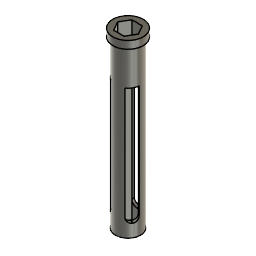
ALL+COMPONENTS+TOGETHER (Autodesk Fusion 360 archive; units mm, degrees)
design "pen holder"
part number: 2025-11-26-14-12-30-338
Autodesk Fusion 360 part; units mm, degrees
note: some values were not read from the file. Set by a fixed rule: which face or edge a step refers to.
sketch "Sketch1" plane through (0, 0, 0) normal (0, 0, 1) x (1, 0, 0)
  circle A0 centre (0, 0) radius 4.9
  line L0 (1.7696, -3.2108) -> (3.6654, -0.0729)
  line L1 (3.6654, -0.0729) -> (1.8959, 3.1379)
  line L2 (1.8959, 3.1379) -> (-1.7696, 3.2108)
  line L3 (-1.7696, 3.2108) -> (-3.6654, 0.0729)
  line L4 (-3.6654, 0.0729) -> (-1.8959, -3.1379)
  line L5 (-1.8959, -3.1379) -> (1.7696, -3.2108)
  dimension "d1" = 9.8
  dimension "d2" = 3.175
  constraint coincident A0.centre origin
  measures "d1" diameter of A0
  measures "d2" distance of A0.centre L5
extrude "Extrude1" add sketch "Sketch1" along normal blind 20 makes body 1
sketch "Sketch2" plane through (0, 0, 20) normal (0, 0, 1) x (-1, 0, 0)
  line L0 (-1.7696, 3.2108) -> (1.8959, 3.1379)
  line L1 (1.8959, 3.1379) -> (3.6654, -0.0729)
  line L2 (3.6654, -0.0729) -> (1.7696, -3.2108)
  line L3 (1.7696, -3.2108) -> (-1.8959, -3.1379)
  line L4 (-1.8959, -3.1379) -> (-3.6654, 0.0729)
  line L5 (-3.6654, 0.0729) -> (-1.7696, 3.2108)
  circle A0 centre (0, 0) radius 4.9
  circle A1 centre (0, 0) radius 6
  dimension "d6" = 12
  constraint concentric A0 A1
  measures "d6" diameter of A1
extrude "Extrude2" add sketch "Sketch2" against normal blind 3 contours A1 bodies 1
sketch "Sketch3" plane through (0, 0, 0) normal (0, 0, -1) x (1, 0, 0)
  line L0 (-1.8959, 3.1379) -> (1.7696, 3.2108)
  line L1 (1.7696, 3.2108) -> (3.6654, 0.0729)
  line L2 (3.6654, 0.0729) -> (1.8959, -3.1379)
  line L3 (1.8959, -3.1379) -> (-1.7696, -3.2108)
  line L4 (-1.7696, -3.2108) -> (-3.6654, -0.0729)
  line L5 (-3.6654, -0.0729) -> (-1.8959, 3.1379)
  circle A0 centre (0, 0) radius 4.9
sketch "Sketch4" plane through (0, 0, 20) normal (0, 0, 1) x (-1, 0, 0)
  circle A0 centre (0, 0) radius 6
  line L0 (-1.7696, 3.2108) -> (1.8959, 3.1379)
  line L1 (1.8959, 3.1379) -> (3.6654, -0.0729)
  line L2 (3.6654, -0.0729) -> (1.7696, -3.2108)
  line L3 (1.7696, -3.2108) -> (-1.8959, -3.1379)
  line L4 (-1.8959, -3.1379) -> (-3.6654, 0.0729)
  line L5 (-3.6654, 0.0729) -> (-1.7696, 3.2108)
  circle A1 centre (0, 0) radius 6
  line L6 (-2.0188, 3.5685) -> (-4.0998, 0.0359)
  line L7 (-4.0998, 0.0359) -> (-2.081, -3.5326)
  line L8 (-2.081, -3.5326) -> (2.0188, -3.5685)
  line L9 (2.0188, -3.5685) -> (4.0998, -0.0359)
  line L10 (4.0998, -0.0359) -> (2.081, 3.5326)
  line L11 (2.081, 3.5326) -> (-2.0188, 3.5685)
  dimension "d9" = 4.1
  constraint coincident A0.centre A1.centre
  measures "d9" distance of L6.start A0.centre
extrude "Extrude3" cut sketch "Sketch4" against normal blind 26 contours L6 L7 L8 L9 L10 L11 bodies 1
extrude "Extrude4" add 1 faces at (-0.1428, -3.9958, 0) along direction (0, 0, -1) blind 118 on bodies 1 bodies 1
extrude "Extrude5" cut 1 faces at (-0.1428, -3.9958, -118) along direction (0, 0, 1) blind 7 on bodies 1 bodies 1
extrude "Extrude6" cut 1 faces at (-0.1428, -3.9958, -111) along direction (0, 0, 1) blind 80 on bodies 1 bodies 1
sketch "Sketch5" plane through (0, 0, -31) normal (0, 0, -1) x (1, 0, 0)
  line L0 (2.0188, 3.5685) -> (4.0998, 0.0359)
  line L1 (4.0998, 0.0359) -> (2.081, -3.5326)
  line L2 (2.081, -3.5326) -> (-2.0188, -3.5685)
  line L3 (-2.0188, -3.5685) -> (-4.0998, -0.0359)
  line L4 (-4.0998, -0.0359) -> (-2.081, 3.5326)
  line L5 (-2.081, 3.5326) -> (2.0188, 3.5685)
  circle A0 centre (0, 0) radius 4.9
  circle A1 centre (0, 0) radius 4.9
  circle A2 centre (0, 0) radius 4.95
  dimension "d18" = 9.9
  constraint concentric A1 A2
  measures "d18" diameter of A2
extrude "Extrude7" add sketch "Sketch5" against normal blind 48 contours A2 bodies 1
extrude "Extrude8" add 1 faces at (3.5469, 1.8815, -31) along direction (0, 0, -1) blind 10 on bodies 1 bodies 1
ref_plane "WorkPlane1" through (0, 0, -37) normal (0, 0, -1) x (-1, 0, 0)
sketch "Sketch6" plane through (0, 0, -37) normal (0, 0, -1) x (-1, 0, 0)
  circle A0 centre (0, 0) radius 4.95
  line L0 (-2.0188, -3.5685) -> (-4.0998, -0.0359)
  line L1 (-4.0998, -0.0359) -> (-2.081, 3.5326)
  line L2 (-2.081, 3.5326) -> (2.0188, 3.5685)
  line L3 (2.0188, 3.5685) -> (4.0998, 0.0359)
  line L4 (4.0998, 0.0359) -> (2.081, -3.5326)
  line L5 (2.081, -3.5326) -> (-2.0188, -3.5685)
  line L6 (-2.081, 3.5326) -> (-2.0894, 4.4874)
  line L7 (2.0188, 3.5685) -> (2.0105, 4.5233)
  line L8 (4.0998, 0.0359) -> (4.9309, -0.4343)
  line L9 (2.081, -3.5326) -> (2.9121, -4.0028)
  line L10 (-2.0188, -3.5685) -> (-2.8416, -4.0532)
  line L11 (-4.0998, -0.0359) -> (-4.9226, -0.5205)
  line L12 (4.0998, 0.0359) -> (2.081, -3.5326)
  line L13 (2.081, -3.5326) -> (-2.0188, -3.5685)
  line L14 (2.0188, 3.5685) -> (4.0998, 0.0359)
  line L15 (-2.081, 3.5326) -> (2.0188, 3.5685)
  line L16 (-4.0998, -0.0359) -> (-2.081, 3.5326)
  line L17 (-2.0188, -3.5685) -> (-4.0998, -0.0359)
  circle A1 centre (0, 0) radius 4.95
  constraint coincident L1.end L2.start
  constraint coincident A0 L6.end
  constraint perpendicular L2 L6
  constraint coincident L2.end L3.start
  constraint coincident A0 L7.end
  constraint perpendicular L2 L7
  constraint coincident L3.end L4.start
  constraint coincident A0 L8.end
  constraint perpendicular L4 L8
  constraint coincident L4.end L5.start
  constraint coincident A0 L9.end
  constraint perpendicular L4 L9
  constraint coincident L0.start L5.end
  constraint coincident A0 L10.end
  constraint perpendicular L0 L10
  constraint coincident L0.end L1.start
  constraint coincident A0 L11.end
  constraint perpendicular L0 L11
split "Split1" by plane through (0, 0, -37) normal (0, 0, -1) bodies 1 makes body 2 at (4.9254, -0.4929, -38.3333)
extrude "Extrude9" cut sketch "Sketch6" against normal blind 40 contours A0 L2 L6 L7 L15 A1 | A0 L4 L8 L9 L12 A1 | A0 L0 L10 L11 L17 A1 bodies 1
move_body "Move1" bodies 2 to x (1, 0, 0) y (0, 1, 0) z (0, 0, 1) at (0, 0, -50)
extrude "Extrude10" add 3 faces at (0.0785, -4.0141, -37) (-3.4002, 2.1348, -37) (3.4516, 2.0525, -37) along direction (0, 0, -1) blind 5 on bodies 1 bodies 1
extrude "Extrude11" add 1 faces at (3.5469, 1.8815, -91) along direction (0, 0, -1) blind 1 on bodies 2 bodies 2
extrude "Extrude12" add 3 faces at (3.5489, 1.8772, -42) (0.0785, -4.0141, -42) (-3.4002, 2.1348, -42) along direction (0, 0, -1) blind 1 on bodies 1 bodies 1
move_body "Align1" bodies 1 to x (1, 0, 0) y (0, 1, 0) z (0, 0, 1) at (0, 0, -44)
combine "Combine1" operation add target body 2 tool bodies 1
fillet "Fillet1" radius 2 2 edges at (4.5112, -0.2782, -87) (2.4302, -3.8108, -87) on bodies 2
fillet "Fillet2" radius 2 4 edges at (-2.0147, 4.0459, -87) (2.0852, 4.01, -87) (-4.5154, -0.1992, -87) (-2.4965, -3.7677, -87) on bodies 2

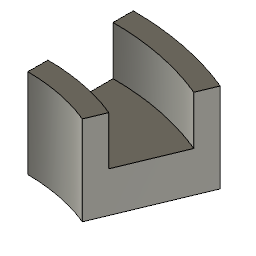
design "legs4"
part number: 2025-11-26-13-44-24-886
Autodesk Fusion 360 part; units mm, degrees
sketch "Sketch1" plane through (0, 0, 0) normal (0, 0, 1) x (1, 0, 0)
  circle A0 centre (0, 0) radius 48.975
  circle A1 centre (0, 0) radius 65.025
  circle A2 centre (0, 0) radius 70.025
  circle A3 centre (0, 0) radius 43.975
  dimension "d7" = 5
  dimension "d9" = -5
extrude "Extrude1" add sketch "Sketch1" along normal blind 12 makes body 1 at (48.9141, -2.4412, 8) makes body 2 at (69.938, -3.4905, 8)
sketch "Sketch2" plane through (0, 0, 0) normal (0, 0, 1) x (1, 0, 0)
  circle A0 centre (0, 0) radius 70
  constraint coincident A0.centre origin
extrude "Extrude2" add sketch "Sketch2" against normal blind 10 bodies 1 2
delete_face "DeleteFace1" 1 faces at (-13.2067, 6.36, 0) on bodies 1
split "Split1" by plane through (0, 0, 0) normal (1, 0, 0) bodies 1 makes body 3 at (60.9383, -5.4068, -10)
delete_body "RemoveBody1" bodies 3
move_body "Move1" bodies 1 to x (0.92388, -0.382683, 0) y (0.382683, 0.92388, 0) z (0, 0, 1) at (0, 0, 0)
split "Split2" by plane through (0, 0, 0) normal (1, 0, 0) bodies 1 makes body 4 at (12.8786, 59.8308, -10)
delete_body "RemoveBody2" bodies 1
equation "d8 = 5.00 mm"
equation "d9 = -d8"

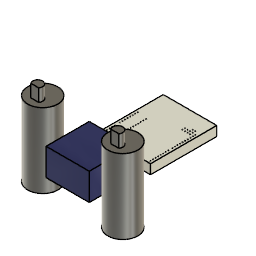
design "elec pieces"
part number: 2025-10-21-14-38-55-580
part number: 2025-10-21-14-53-44-347
part number: 2025-10-21-15-16-38-518
part number: 2025-10-21-15-29-22-499
Autodesk Fusion 360 part; units mm, degrees
sketch "Sketch1" plane through (0, 0, 0) normal (0, 0, 1) x (1, 0, 0)
sketch "Sketch2" plane through (0, -1.65, 0) normal (0, -1, 0) x (1, 0, 0)
  line L0 (0, -66.04) -> (0, 0)
  line L1 (0, 0) -> (-53.34, 0)
  line L2 (-53.34, 0) -> (-53.34, -66.04)
  line L3 (-53.34, -66.04) -> (-40.386, -66.04)
  line L4 (-40.386, -66.04) -> (-37.846, -68.58)
  line L5 (-37.846, -68.58) -> (-5.08, -68.58)
  line L6 (-5.08, -68.58) -> (-2.54, -66.04)
  line L7 (-2.54, -66.04) -> (0, -66.04)
  circle A0 centre (-2.54, -33.02) radius 0.4
  circle A1 centre (-2.54, -35.56) radius 0.4
  circle A2 centre (-2.54, -38.1) radius 0.4
  circle A3 centre (-2.54, -40.64) radius 0.4
  circle A4 centre (-2.54, -43.18) radius 0.4
  circle A5 centre (-2.54, -45.72) radius 0.4
  circle A6 centre (-2.54, -50.8) radius 0.4
  circle A7 centre (-2.54, -53.34) radius 0.4
  circle A8 centre (-2.54, -55.88) radius 0.4
  circle A9 centre (-2.54, -58.42) radius 0.4
  circle A10 centre (-2.54, -60.96) radius 0.4
  circle A11 centre (-2.54, -63.5) radius 0.4
  circle A12 centre (-50.8, -23.876) radius 0.4
  circle A13 centre (-50.8, -26.416) radius 0.4
  circle A14 centre (-50.8, -28.956) radius 0.4
  circle A15 centre (-50.8, -31.496) radius 0.4
  circle A16 centre (-50.8, -34.036) radius 0.4
  circle A17 centre (-50.8, -36.576) radius 0.4
  circle A18 centre (-50.8, -39.116) radius 0.4
  circle A19 centre (-50.8, -41.656) radius 0.4
  circle A20 centre (-50.8, -50.8) radius 0.4
  circle A21 centre (-50.8, -53.34) radius 0.4
  circle A22 centre (-50.8, -55.88) radius 0.4
  circle A23 centre (-50.8, -58.42) radius 0.4
  circle A24 centre (-50.8, -60.96) radius 0.4
  circle A25 centre (-50.8, -63.5) radius 0.4
  circle A26 centre (-12.573, -62.865) radius 0.4
  circle A27 centre (-20.193, -62.865) radius 0.4
  circle A28 centre (-12.573, -60.325) radius 0.4
  circle A29 centre (-20.193, -60.325) radius 0.4
  circle A30 centre (-12.573, -57.785) radius 0.4
  circle A31 centre (-20.193, -57.785) radius 0.4
  circle A32 centre (-12.573, -55.245) radius 0.4
  circle A33 centre (-20.193, -55.245) radius 0.4
  circle A34 centre (-12.573, -52.705) radius 0.4
  circle A35 centre (-20.193, -52.705) radius 0.4
  circle A36 centre (-12.573, -50.165) radius 0.4
  circle A37 centre (-20.193, -50.165) radius 0.4
  circle A38 centre (-12.573, -47.625) radius 0.4
  circle A39 centre (-20.193, -47.625) radius 0.4
  circle A40 centre (-12.573, -45.085) radius 0.4
  circle A41 centre (-20.193, -45.085) radius 0.4
  circle A42 centre (-12.573, -42.545) radius 0.4
  circle A43 centre (-20.193, -42.545) radius 0.4
  circle A44 centre (-12.573, -40.005) radius 0.4
  circle A45 centre (-20.193, -40.005) radius 0.4
  circle A46 centre (-12.573, -37.465) radius 0.4
  circle A47 centre (-20.193, -37.465) radius 0.4
  circle A48 centre (-12.573, -34.925) radius 0.4
  circle A49 centre (-20.193, -34.925) radius 0.4
  circle A50 centre (-12.573, -32.385) radius 0.4
  circle A51 centre (-20.193, -32.385) radius 0.4
  circle A52 centre (-12.573, -29.845) radius 0.4
  circle A53 centre (-20.193, -29.845) radius 0.4
  circle A54 centre (-26.162, -16.383) radius 0.5
  circle A55 centre (-26.162, -21.463) radius 0.5
  circle A56 centre (-39.878, -18.288) radius 0.4
  circle A57 centre (-39.878, -20.828) radius 0.4
  circle A58 centre (-42.418, -20.828) radius 0.4
  circle A59 centre (-42.418, -18.288) radius 0.4
  circle A60 centre (-44.958, -15.748) radius 0.4
  circle A61 centre (-44.958, -18.288) radius 0.4
  circle A62 centre (-44.958, -20.828) radius 0.4
  circle A63 centre (-47.498, -20.828) radius 0.4
  circle A64 centre (-47.498, -18.288) radius 0.4
  circle A65 centre (-47.498, -15.748) radius 0.4
  circle A66 centre (-30.43, -63.64) radius 0.4
  circle A67 centre (-27.89, -63.64) radius 0.4
  circle A68 centre (-25.35, -63.64) radius 0.4
  circle A69 centre (-25.35, -66.18) radius 0.4
  circle A70 centre (-27.89, -66.18) radius 0.4
  circle A71 centre (-30.43, -66.18) radius 0.4
  circle A72 centre (-50.8, -48.26) radius 0.4
  circle A73 centre (-50.8, -21.336) radius 0.4
  circle A74 centre (-50.8, -45.72) radius 0.4
  circle A75 centre (-2.54, -30.48) radius 0.4
  circle A76 centre (-50.8, -18.796) radius 0.4
  circle A77 centre (-2.54, -27.94) radius 0.4
  circle A78 centre (-50.8, -15.24) radius 1.5875
  circle A79 centre (-2.54, -13.97) radius 1.5875
  circle A80 centre (-35.56, -66.04) radius 1.5875
  circle A81 centre (-7.62, -66.04) radius 1.5875
  line L8 (-53.34, 0) -> (0, 0)
  line L9 (0, 0) -> (0, -66.04)
  line L10 (0, -66.04) -> (-53.34, -66.04)
  line L11 (-53.34, -66.04) -> (-53.34, 0)
  constraint horizontal L8
  constraint vertical L9
  constraint horizontal L10
  constraint vertical L11
  constraint coincident L0.start L7.end
  constraint coincident L1.end L2.start
extrude "Extrude1" add sketch "Sketch2" along normal blind 9.55 contours L0 L1 L2 L3 L7 A69 A70 A71 A80 A81 L8 L9 L10 L11 | A81 L10 | A80 L10 | A78 | A79 picked at (-7.5022, -65.5241) picked at (-35.4422, -65.5241) makes body 1 in component "Breadboard"
delete_face "DeleteFace1" 15 faces at (-25.6775, -8.0167, -21.5864) (-25.8129, -8.0167, -16.0251) (-20.183, -8.0167, -29.4451) (-19.7935, -8.0167, -32.4049) (-19.7935, -8.0167, -34.9449) (-19.7935, -8.0167, -37.4849) (-19.7935, -8.0167, -40.0249) (-19.7935, -8.0167, -42.5649) (-19.7935, -8.0167, -45.1049) (-19.7935, -8.0167, -47.6449) (-19.7935, -8.0167, -50.1849) (-19.7935, -8.0167, -52.7249) (-19.7935, -8.0167, -55.2649) (-19.7935, -8.0167, -57.8049) (-19.7935, -8.0167, -60.3449) on bodies 1 in component "Breadboard"
delete_face "DeleteFace2" 9 faces at (-25.0188, -8.0167, -65.9556) (-28.2212, -4.8333, -65.9556) (-30.7612, -4.8333, -65.9556) (-30.0305, -8.0167, -63.6599) (-27.4905, -8.0167, -63.6599) (-24.9505, -8.0167, -63.6599) (-19.7935, -8.0167, -62.8849) (-12.9143, -8.0167, -63.0736) (-12.9143, -8.0167, -60.5336) on bodies 1 in component "Breadboard"
sketch "Sketch3" plane through (0, 0, 0) normal (0, 1, 0) x (1, 0, 0)
  circle A0 centre (15, -15) radius 15
  dimension "d3" = 30
  measures "d3" diameter of A0
extrude "Extrude1'" add sketch "Sketch3" along normal blind 74.1 separate body makes body 2
sketch "Sketch4" plane through (0, 74.1, 0) normal (0, 1, 0) x (-1, 0, 0)
  circle A0 centre (-15, 15) radius 15
  circle A1 centre (-15, 20) radius 5
  line L0 (-30, 15) -> (0, 15) construction
  line L1 (-15, 30) -> (-15, 0) construction
  line L2 (-29.1421, 20) -> (-0.8579, 20) construction
  line L3 (-24.0791, 20) -> (-24.0791, 15) construction
  line L4 (-19, 23) -> (-11, 23)
  dimension "d6" = 10
  dimension "d7" = 5
  constraint coincident A0 L0.start
  constraint coincident A0 L0.end
  constraint horizontal L0
  constraint coincident A0 L1.start
  constraint coincident A0 L1.end
  constraint perpendicular L0 L1
  constraint coincident A0 L2.start
  constraint coincident A0 L2.end
  constraint perpendicular L1 L2
  constraint coincident L2 L3.start
  constraint perpendicular L0 L3
  constraint coincident L0 L3.end
  constraint coincident A1.centre L1
  constraint coincident A1.centre L2
  constraint coincident A1 L4.start
  constraint coincident A1 L4.end
  constraint perpendicular L1 L4
  measures "d6" diameter of A1
  measures "d7" distance of L3.start L3.end
extrude "Extrude2" add sketch "Sketch4" along normal blind 12.5 contours A1 L4 picked at (-15.5407, 20.0355) bodies 2
copy_body "Body->Comp1" bodies 2 removing the originals makes body 3 in component "Motors"
sketch "Sketch5" plane through (0, 0, 0) normal (0, 1, 0) x (1, 0, 0)
  line L0 (0, -25) -> (-43, -25)
  line L1 (-43, -25) -> (-43, -68)
  line L2 (-43, -68) -> (0, -68)
  line L3 (0, -68) -> (0, -25)
  dimension "d10" = 43
  dimension "d11" = 43
  constraint horizontal L0
  constraint vertical L1
  constraint horizontal L2
  constraint vertical L3
  measures "d10" distance of L0.start L0.end
  measures "d11" distance of L0.start L2.end
extrude "Extrude3" add sketch "Sketch5" along normal blind 27 separate body makes body 4
copy_body "Body->Comp2" bodies 4 removing the originals makes body 5 in component "H-Bridge Motor Driver"
component "Breadboard" placed x (1, 0, 0) y (0, 1, 0) z (0, 0, 1) at (0, 11, 0)
component "Motors" placed x (1, 0, 0) y (0, 1, 0) z (0, 0, 1) at (9.7018, 0.2853, 0)
component "Motors" placed x (1, 0, 0) y (0, 1, 0) z (0, 0, 1) at (-90, 0, 0)
component "H-Bridge Motor Driver" placed x (1, 0, 0) y (0, 1, 0) z (0, 0, 1) at (0, 0, 0)

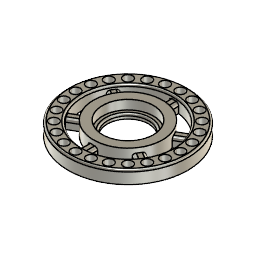
design "base bottom bearing"
part number: 2025-10-22-14-24-42-965
Autodesk Fusion 360 part; units mm, degrees
sketch "Sketch2" plane through (0, 0, 0) normal (0, 0, 1) x (1, 0, 0)
  circle A0 centre (0, 0) radius 65
  dimension "d1" = 130
  constraint coincident A0.centre origin
  measures "d1" diameter of A0
extrude "Extrude1" add sketch "Sketch2" along normal blind 20
sketch "Sketch3" plane through (0, 0, 20) normal (0, 0, 1) x (-1, 0, 0)
  circle A0 centre (0, 0) radius 65
  circle A1 centre (0, 0) radius 27.6
  circle A2 centre (0, 0) radius 49
  circle A3 centre (0, -57) radius 5
  line L0 (0, -65) -> (0, -49) construction
  circle A4 centre (14.7527, -55.0578) radius 5
  circle A5 centre (28.5, -49.3634) radius 5
  circle A6 centre (40.3051, -40.3051) radius 5
  circle A7 centre (49.3634, -28.5) radius 5
  circle A8 centre (55.0578, -14.7527) radius 5
  circle A9 centre (57, 0) radius 5
  circle A10 centre (55.0578, 14.7527) radius 5
  circle A11 centre (49.3634, 28.5) radius 5
  circle A12 centre (40.3051, 40.3051) radius 5
  circle A13 centre (28.5, 49.3634) radius 5
  circle A14 centre (14.7527, 55.0578) radius 5
  circle A15 centre (0, 57) radius 5
  circle A16 centre (-14.7527, 55.0578) radius 5
  circle A17 centre (-28.5, 49.3634) radius 5
  circle A18 centre (-40.3051, 40.3051) radius 5
  circle A19 centre (-49.3634, 28.5) radius 5
  circle A20 centre (-55.0578, 14.7527) radius 5
  circle A21 centre (-57, 0) radius 5
  circle A22 centre (-55.0578, -14.7527) radius 5
  circle A23 centre (-49.3634, -28.5) radius 5
  circle A24 centre (-40.3051, -40.3051) radius 5
  circle A25 centre (-28.5, -49.3634) radius 5
  circle A26 centre (-14.7527, -55.0578) radius 5
  circle A27 centre (0, 0) radius 22.5
  circle A28 centre (0, 0) radius 37.5
  line L1 (4.221, -37.2617) -> (4.221, -48.8179)
  line L2 (-6.4986, -36.9326) -> (-6.4986, -48.5672)
  line L3 (34.3801, -14.9753) -> (44.388, -20.7534)
  line L4 (28.7353, -24.0943) -> (38.8111, -29.9115)
  line L5 (30.1591, 22.2864) -> (40.167, 28.0644)
  line L6 (35.2339, 12.8384) -> (45.3097, 18.6556)
  line L7 (-4.221, 37.2617) -> (-4.221, 48.8179)
  line L8 (6.4986, 36.9326) -> (6.4986, 48.5672)
  line L9 (-34.3801, 14.9753) -> (-44.388, 20.7534)
  line L10 (-28.7353, 24.0943) -> (-38.8111, 29.9115)
  line L11 (-30.1591, -22.2864) -> (-40.167, -28.0644)
  line L12 (-35.2339, -12.8384) -> (-45.3097, -18.6556)
  dimension "d4" = 55.2
  dimension "d6" = 98
  dimension "d7" = 10
  dimension "d34" = 45
  dimension "d39" = 75
  dimension "d41" = 360
  constraint coincident A0.centre A1.centre
  constraint coincident A0 L0.start
  constraint coincident A2 L0.end
  constraint vertical L0
  constraint coincident A3.centre L0
  constraint concentric A2 A28
  constraint coincident A28 L1.start
  constraint coincident A2 L1.end
  constraint coincident A2 L2.end
  constraint vertical L2
  constraint parallel L1 L2
  constraint coincident A28 L2.start
  measures "d4" diameter of A1
  measures "d6" diameter of A2
  measures "d7" diameter of A3
  measures "d34" diameter of A27
  measures "d39" diameter of A28
extrude "Extrude11" cut sketch "Sketch3" against normal blind 60 contours A27
extrude "Extrude12" cut sketch "Sketch3" against normal blind 15 contours A1
extrude "Extrude13" cut sketch "Sketch3" against normal blind 35 contours A2 A28 L3 L6 | A2 A28 L5 L8 | A2 A28 L1 L4 | A2 A28 L7 L10 | A2 A28 L2 L11 | A2 A28 L9 L12
extrude "Extrude14" cut sketch "Sketch3" against normal blind 10 contours A2 A28 L5 L6 | A2 A28 L3 L4 | A2 A28 L7 L8 | A2 A28 L1 L2 | A2 A28 L9 L10 | A2 A28 L11 L12
extrude "Extrude15" cut sketch "Sketch3" against normal blind 16 contours A3 | A4 | A5 | A6 | A7 | A8 | A9 | A10 | A11 | A12 | A13 | A14 | A15 | A16 | A17 | A18 | A19 | A20 | A21 | A22 | A23 | A24 | A25 | A26
fillet "Fillet2" radius 3 12 edges at (6.4986, 42.7499, 10) (-4.221, 43.0398, 10) (-39.384, 17.8644, 10) (-33.7732, 27.0029, 10) (-35.163, -25.1754, 10) (-40.2718, -15.747, 10) (-6.4986, -42.7499, 10) (4.221, -43.0398, 10) (33.7732, -27.0029, 10) (39.384, -17.8644, 10) (40.2718, 15.747, 10) (35.163, 25.1754, 10)
fillet "Fillet4" radius 2 1 edges at (20.9774, 8.1363, 5)
extrude "Extrude16" cut 1 faces at (-31.0092, -14.2533, 20) along direction (0, 0, -1) blind 5
extrude "Extrude17" cut 1 faces at (-60.4253, 8.3952, 20) along direction (0, 0, -1) blind 5
extrude "Extrude18" cut 1 faces at (-60.4253, 8.3952, 15) along direction (0, 0, -1) blind 1
fillet "Fillet5" radius 2 2 edges at (-60.6013, 23.505, 14) (45.684, 17.7192, 14)
